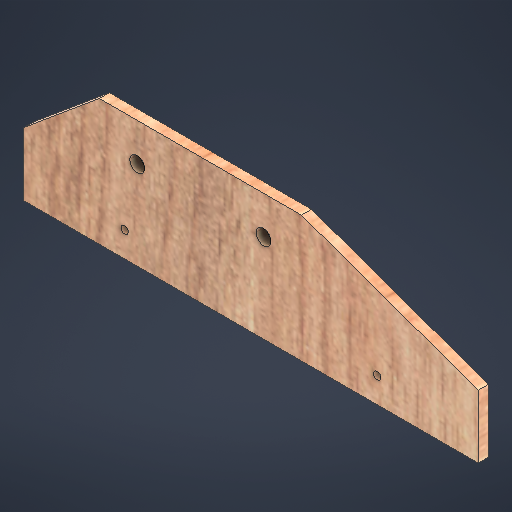
# Autodesk Inventor part: Trup
Saved by Autodesk Inventor 2026 (Build 300175050, 175E)
## iProperties
Created: 2026-03-01
Part Number: Trup
Material: Dřevo (Bříza)
Document SubType Name: Modeling
Designer: marti
Density: 0.55 g/cm^3
Appearance: Bříza – přírodní leštěná
Author: marti
Autodesk Inventor part; units mm, degrees
ref_plane "YZ Plane" through (0, 0, 0) normal (1, 0, 0) x (0, 1, 0)
ref_plane "XZ Plane" through (0, 0, 0) normal (0, 1, 0) x (-1, 0, 0)
ref_plane "XY Plane" through (0, 0, 0) normal (0, 0, 1) x (1, 0, 0)
sketch "Náčrt1" plane through (0, 0, 0) normal (0, 0, 1) x (1, 0, 0)
  line L0 (-50, 25) -> (30, 25)
  line L1 (36.6643, -25) -> (-87.5, -25)
  line L2 (30, 25) -> (100, 0)
  line L3 (100, 0) -> (100, -25)
  line L4 (100, -25) -> (36.6643, -25)
  line L5 (-125, 0) -> (137.5, 0) projected
  line L6 (0, 35) -> (0, -35) projected
  line L7 (-50, 25) -> (-80, 0)
  line L8 (-80, 0) -> (-80, -25)
  line L9 (-80, -25) -> (-87.5, -25)
  point P0 (0, 0)
  point P1 (-35, 10)
  point P2 (15, 10)
  dimension "d0" = 50
  dimension "d2" = 80
  dimension "d3" = 25
  dimension "d4" = 50
  dimension "d6" = 15
  dimension "d16" = 70
  dimension "d17" = 30
  dimension "d18" = 25
  dimension "d19" = 50
  dimension "d20" = 35
  dimension "d21" = 25
  dimension "d22" = 25
  constraints: 16 end point, 2 vertical, 1 collinear, 1 horizontal, 1 parallel, 1 perpendicular, 1 other
  measures "d0" distance between parallel lines of L1 L0
  measures "d2" distance of L0.start L0.end
  measures "d3" distance of L2.end L3.end
  measures "d4" distance of point (15, 10) point (-35, 10)
  measures "d6" distance from line of L0 point (-35, 10)
  measures "d16" distance from line of L3 L0.end
  measures "d17" distance from line of L8 L0.start
  measures "d18" distance of L8.end L7.end
  measures "d19" distance from line of L6 L0.start
  measures "d20" distance from line of L6 point (-35, 10)
  measures "d21" vertical distance of L0.start L7.end
  measures "d22" vertical distance of L2.end L0.end
extrude "Vysunutí1" add sketch "Náčrt1" along normal mid plane 4
hole "Díra1" at (-35, 10, 0) at (15, 10, 0) direction (0, 0, -1) diameter 6 end through all both
sketch "Náčrt2" plane through (0, 0, 2) normal (0, 0, 1) x (1, 0, 0)
  line L0 (-80, 0) -> (-80, -25) projected
  line L1 (-80, -25) -> (100, -25) projected
  line L2 (100, -25) -> (100, 0) projected
  point P0 (0, 0)
  point P1 (-40, -15)
  point P2 (60, -15)
  dimension "d23" = 40
  dimension "d24" = 10
  dimension "d25" = 40
  dimension "d26" = 10
  measures "d23" distance from line of L0 point (-40, -15)
  measures "d24" distance from line of L1 point (-40, -15)
  measures "d25" distance from line of L2 point (60, -15)
  measures "d26" distance from line of L1 point (60, -15)
hole "Díra2" at (-40, -15, 2) at (60, -15, 2) direction (0, 0, -1) diameter 3 depth 8
